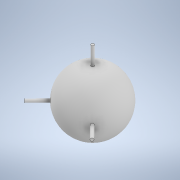
# Autodesk Inventor part: solid bottom ball
Saved by Autodesk Inventor 2022 (Build 260153000, 153)
## iProperties
Created: 2022-03-15
Part Number: solid bottom ball
Material: Generic
Document SubType Name: Modeling
Designer: mogje
Density: 1 g/cm^3
Appearance: Default
Author: mogje
Autodesk Inventor part; units mm, degrees
ref_plane "YZ Plane" through (0, 0, 0) normal (1, 0, 0) x (0, 1, 0)
ref_plane "XZ Plane" through (0, 0, 0) normal (0, 1, 0) x (-1, 0, 0)
ref_plane "XY Plane" through (0, 0, 0) normal (0, 0, 1) x (1, 0, 0)
sketch "Sketch1" plane through (0, 0, 0) normal (0, 1, 0) x (-1, 0, 0)
  arc A0 (-31.75, 0) -> (31.75, 0) centre (0, 0) ccw
  line L0 (0, 0) -> (-31.75, 0) construction
  line L1 (0, 0) -> (31.75, 0) construction
  line L2 (31.75, 0) -> (-31.75, 0)
  dimension "d0" = 31.75
  dimension "d1" = 180
  constraints: 6 end point, 2 point on circle, 1 centre point, 1 coincident
  measures "d0" radius of A0
  measures "d1" angle of L0 L1
revolve "Revolution1" add sketch "Sketch1" angle 360 about axis through (0, 0, 0) along (1, 0, 0)
sketch "Sketch2" plane through (0, 0, 0) normal (0, 1, 0) x (-1, 0, 0)
  circle A0 centre (0, 0) radius 31.75 projected
  circle A1 centre (0, 0) radius 31.75 projected
  line L0 (30.7725, 7.8175) -> (7.1862, 30.9261)
  circle A2 centre (0, 0) radius 31.75 projected
  line L1 (0, 31.75) -> (0, -31.75)
  circle A3 centre (0, 0) radius 31.75 projected
  line L2 (-30.7725, 7.8175) -> (-7.1862, 30.9261)
  arc A4 (7.1862, 30.9261) -> (-7.1862, 30.9261) centre (0, 0) ccw
  arc A5 (-30.7725, 7.8175) -> (30.7725, 7.8175) centre (0, 0) ccw
  constraints: 6 end point, 4 point on circle, 2 centre point, 2 symmetric about line, 2 vertical alignment, 1 coincident, 1 vertical, 2 other
extrude "Extrusion1" cut sketch "Sketch2" along normal blind 38.1 and the other way blind 29.21 contours A0 L1 L0 | A0 L2 L1 keep common part
sketch "Sketch3" plane through (0, 0, 0) normal (1, 0, 0) x (0, 1, 0)
  arc A0 (27.1198, 16.51) -> (27.1198, -16.51) centre (0, 0) ccw
  line L0 (27.1198, 16.51) -> (27.1198, -16.51)
  dimension "d9" = 33.02
  dimension "d10" = 63.5
  constraints: 2 end point, 2 point on circle, 1 centre point, 1 coincident, 1 vertical
  measures "d9" distance of L0.start L0.end
  measures "d10" diameter of A0
extrude "Extrusion2" cut sketch "Sketch3" along normal mid plane 101.6 keep common part
sketch "Sketch4" plane through (18.9794, 0, 19.3718) normal (0.6998, 0, 0.7143) x (0.7143, 0, -0.6998)
  circle A0 centre (0, 0) radius 1.5875
  constraints: 1 centre point, 1 coincident
extrude "Extrusion3" add sketch "Sketch4" along normal blind 23.6728
sketch "Sketch7" plane through (0, 27.1198, 0) normal (0, 1, 0) x (1, 0, 0)
  circle A0 centre (0, 0) radius 1.5875
  dimension "d18" = 3.175
  constraints: 1 centre point, 1 coincident
  measures "d18" diameter of A0
extrude "Extrusion4" add sketch "Sketch7" along normal blind 23.6728
sketch "Sketch8" plane through (-18.9794, 0, 19.3718) normal (-0.6998, 0, 0.7143) x (0.7143, 0, 0.6998)
  circle A0 centre (0, 0) radius 1.5875
  dimension "d21" = 3.175
  constraints: 1 centre point, 1 coincident
  measures "d21" diameter of A0
extrude "Extrusion5" add sketch "Sketch8" along normal blind 23.6728
sketch "Sketch9" plane through (0, 0, 0) normal (0, 1, 0) x (-1, 0, 0)
  circle A0 centre (0, 0) radius 1.5875 projected
  arc A1 (-30.7725, 7.8175) -> (-7.1862, 30.9261) centre (0, 0) ccw projected
  arc A2 (0, 31.75) -> (0, -31.75) centre (0, 0) ccw
  line L0 (0, -31.75) -> (0, 31.75)
  point P0 (0, 1.5875)
  point P1 (-7.1862, 30.9261)
  point P2 (-30.7725, 7.8175)
  point P3 (0, -1.5875)
  constraints: 4 point on circle, 2 end point, 1 centre point, 1 coincident, 1 vertical
sketch "Sketch10" plane through (0, -29.21, 0) normal (0, -1, 0) x (1, 0, 0)
  circle A0 centre (0, 0) radius 1.5875 projected
  circle A1 centre (0, 0) radius 12.4434
  point P0 (0, 0)
  constraints: 1 centre point, 1 coincident
revolve "Revolution2" add sketch "Sketch9" angle 360 about axis through (0, 0, -31.75) along (0, 0, 1) contours A0 L0 A1 A2
extrude "Extrusion6" cut sketch "Sketch10" along normal blind 101.6 contours A0 | A1
body "Solid1"
